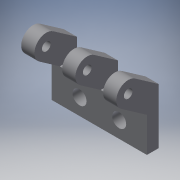
# Autodesk Inventor part: xy 아이들러
Saved by Autodesk Inventor 2018 (Build 220112000, 112)
## iProperties
Created: 2019-01-21
Part Number: xy 아이들러
Material: Generic
Document SubType Name: Modeling
Designer: User
Density: 1 g/cm^3
Appearance: Default
Author: User
Autodesk Inventor part; units mm, degrees
ref_plane "YZ Plane" through (0, 0, 0) normal (1, 0, 0) x (0, 1, 0)
ref_plane "XZ Plane" through (0, 0, 0) normal (0, 1, 0) x (-1, 0, 0)
ref_plane "XY Plane" through (0, 0, 0) normal (0, 0, 1) x (1, 0, 0)
sketch "스케치1" plane through (0, 0, 0) normal (1, 0, 0) x (0, 1, 0)
  circle A0 centre (0, 0) radius 1.65
  line L0 (-23.6101, -11.5918) -> (-23.6101, -7.0918)
  arc A1 (3.6862, -2.5811) -> (-3.6862, 2.5811) centre (0, 0) ccw
  line L1 (-3.6862, 2.5811) -> (-10.4592, -7.0918)
  line L2 (-10.4592, -7.0918) -> (-23.6101, -7.0918)
  line L3 (3.6862, -2.5811) -> (-2.6232, -11.5918)
  line L4 (-2.6232, -11.5918) -> (-23.6101, -11.5918)
  line L5 (-10.4592, -7.0918) -> (-9.0498, -7.0918)
  line L6 (-9.0498, -7.0918) -> (-9.0498, -11.5918)
  dimension "d5" = 4.5
  constraints: 14 end point, 3 coincident, 3 horizontal, 2 centre point, 2 point on circle, 1 perpendicular, 1 point on line, 1 vertical
  measures "d5" distance of L0.start L0.end
extrude "돌출1" add sketch "스케치1" along normal blind 36 contours A0 | L0 L2 L5 L6 L4 | L6 L5 L1 A1 L3 L4
sketch "스케치4" plane through (0, -23.6101, -11.5918) normal (0, 0, -1) x (-1, 0, 0)
  line L0 (-36, 14.5515) -> (-31, 14.5515)
  line L1 (-31, 14.5515) -> (-30, 14.5515)
  line L2 (-30, 14.5515) -> (-21.5, 14.5515)
  line L3 (-21.5, 14.5515) -> (-20.5, 14.5515)
  line L4 (-20.5, 14.5515) -> (-15.5, 14.5515)
  line L5 (-15.5, 14.5515) -> (-14.5, 14.5515)
  line L6 (-14.5, 14.5515) -> (-6, 14.5515)
  line L7 (-6, 14.5515) -> (-5, 14.5515)
  line L8 (-5, 14.5515) -> (0, 14.5515)
  line L9 (-36, 14.5515) -> (-36, 28.1225)
  line L10 (-36, 28.1225) -> (-31, 28.1225)
  line L11 (-31, 28.1225) -> (-31, 14.5515)
  line L12 (-31, 14.5515) -> (-36, 14.5515)
  line L13 (-36, 19.9239) -> (-36, 13.1509) projected
  line L14 (-31, 28.1225) -> (-30, 28.1225)
  line L15 (-30, 28.1225) -> (-30, 14.5515)
  line L16 (-30, 14.5515) -> (-31, 14.5515)
  line L17 (-31, 14.5515) -> (-31, 28.1225)
  line L18 (-30, 28.1225) -> (-21.5, 28.1225)
  line L19 (-21.5, 28.1225) -> (-21.5, 14.5515)
  line L20 (-21.5, 14.5515) -> (-30, 14.5515)
  line L21 (-30, 14.5515) -> (-30, 28.1225)
  line L22 (-21.5, 28.1225) -> (-20.5, 28.1225)
  line L23 (-20.5, 28.1225) -> (-20.5, 14.5515)
  line L24 (-20.5, 14.5515) -> (-21.5, 14.5515)
  line L25 (-21.5, 14.5515) -> (-21.5, 28.1225)
  line L26 (-20.5, 28.1225) -> (-15.5, 28.1225)
  line L27 (-15.5, 28.1225) -> (-15.5, 14.5515)
  line L28 (-15.5, 14.5515) -> (-20.5, 14.5515)
  line L29 (-20.5, 14.5515) -> (-20.5, 28.1225)
  line L30 (-15.5, 28.1225) -> (-14.5, 28.1225)
  line L31 (-14.5, 28.1225) -> (-14.5, 14.5515)
  line L32 (-14.5, 14.5515) -> (-15.5, 14.5515)
  line L33 (-15.5, 14.5515) -> (-15.5, 28.1225)
  line L34 (-14.5, 28.1225) -> (-6, 28.1225)
  line L35 (-6, 28.1225) -> (-6, 14.5515)
  line L36 (-6, 14.5515) -> (-14.5, 14.5515)
  line L37 (-14.5, 14.5515) -> (-14.5, 28.1225)
  line L38 (-6, 28.1225) -> (-5, 28.1225)
  line L39 (-5, 28.1225) -> (-5, 14.5515)
  line L40 (-5, 14.5515) -> (-6, 14.5515)
  line L41 (-6, 14.5515) -> (-6, 28.1225)
  line L42 (-5, 28.1225) -> (0, 28.1225)
  line L43 (0, 28.1225) -> (0, 14.5515)
  line L44 (0, 14.5515) -> (-5, 14.5515)
  line L45 (-5, 14.5515) -> (-5, 28.1225)
  line L46 (-36, 13.1509) -> (-10.5, 13.1509)
  line L47 (0, 13.1509) -> (-36, 13.1509) projected
  line L48 (-18, 13.1509) -> (-18, 6.1509)
  line L49 (-18, 6.1509) -> (-25.5, 6.1509)
  line L50 (-18, 6.1509) -> (-10.5, 6.1509)
  circle A0 centre (-25.5, 6.1509) radius 2.65
  circle A1 centre (-10.5, 6.1509) radius 2.65
  dimension "d17" = 5
  dimension "d18" = 1
  dimension "d19" = 8.5
  dimension "d20" = 1
  dimension "d21" = 5
  dimension "d22" = 1
  dimension "d23" = 8.5
  dimension "d24" = 1
  dimension "d25" = 5
  dimension "d38" = 7
  dimension "d39" = 7.5
  dimension "d40" = 7.5
  dimension "d41" = 5.3
  dimension "d42" = 5.3
  constraints: 98 end point, 18 parallel, 10 perpendicular, 9 horizontal, 2 centre point, 2 coincident, 2 collinear, 1 midpoint, 1 point on line, 1 vertical
  measures "d17" distance of L0.start L0.end
  measures "d18" distance of L0.end L1.end
  measures "d19" distance of L1.end L2.end
  measures "d20" distance of L2.end L3.end
  measures "d21" distance of L3.end L4.end
  measures "d22" distance of L4.end L5.end
  measures "d23" distance of L5.end L6.end
  measures "d24" distance of L6.end L7.end
  measures "d25" distance of L7.end L8.end
  measures "d38" distance of L48.start L48.end
  measures "d39" distance of L48.end L49.end
  measures "d40" distance of L48.end L50.end
  measures "d41" diameter of A0
  measures "d42" diameter of A1
extrude "돌출2" cut sketch "스케치4" against normal blind 18 contours L11 L14 L15 L1 | L15 L18 L19 L2 | L19 L22 L23 L3 | L27 L30 L31 L5 | L31 L34 L35 L6 | L35 L38 L39 L7
extrude "돌출3" cut sketch "스케치1" along normal blind 36 contours A0
extrude "돌출6" cut sketch "스케치4" against normal blind 10 contours A0
extrude "돌출7" cut sketch "스케치4" against normal blind 10 contours A1
